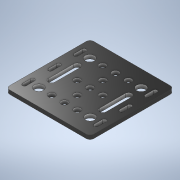
# Autodesk Inventor part: Plataforma
Saved by Autodesk Inventor 2021 (Build 250183000, 183)
## iProperties
Created: 2022-01-21
Part Number: Plataforma
Material: Generic
Document SubType Name: Modeling
Designer: deuts
Density: 1 g/cm^3
Appearance: Default
Author: deuts
Autodesk Inventor part; units mm, degrees
ref_plane "YZ Plane" through (0, 0, 0) normal (1, 0, 0) x (0, 1, 0)
ref_plane "XZ Plane" through (0, 0, 0) normal (0, 1, 0) x (-1, 0, 0)
ref_plane "XY Plane" through (0, 0, 0) normal (0, 0, 1) x (1, 0, 0)
sketch "Sketch1" plane through (0, 0, 0) normal (0, 1, 0) x (-1, 0, 0)
  line L0 (-29.75, 32.75) -> (29.75, 32.75)
  line L1 (32.75, 29.75) -> (32.75, -29.75)
  line L2 (29.75, -32.75) -> (-29.75, -32.75)
  line L3 (-32.75, -29.75) -> (-32.75, 29.75)
  arc A0 (-29.75, 32.75) -> (-32.75, 29.75) centre (-29.75, 29.75) ccw
  arc A1 (-32.75, -29.75) -> (-29.75, -32.75) centre (-29.75, -29.75) ccw
  arc A2 (29.75, -32.75) -> (32.75, -29.75) centre (29.75, -29.75) ccw
  arc A3 (32.75, 29.75) -> (29.75, 32.75) centre (29.75, 29.75) ccw
  arc A4 (29.2, 23.4) -> (26.2, 23.4) centre (27.7, 23.4) ccw
  arc A5 (26.2, 16.9) -> (29.2, 16.9) centre (27.7, 16.9) ccw
  line L4 (29.2, 23.4) -> (29.2, 16.9)
  line L5 (26.2, 23.4) -> (26.2, 16.9)
  arc A6 (29.2, 3.25) -> (26.2, 3.25) centre (27.7, 3.25) ccw
  arc A7 (26.2, -3.25) -> (29.2, -3.25) centre (27.7, -3.25) ccw
  line L6 (29.2, 3.25) -> (29.2, -3.25)
  line L7 (26.2, 3.25) -> (26.2, -3.25)
  circle A8 centre (20, 19.85) radius 3.6
  circle A9 centre (10, 19.85) radius 2.55
  circle A10 centre (0, 19.85) radius 2.55
  circle A11 centre (0, 10) radius 2.55
  circle A12 centre (0, 0) radius 2.55
  circle A13 centre (10, 0) radius 2.55
  arc A14 (22.5, 10) -> (17.5, 10) centre (20, 10) ccw
  arc A15 (17.5, -10) -> (22.5, -10) centre (20, -10) ccw
  line L8 (22.5, 10) -> (22.5, -10)
  line L9 (17.5, 10) -> (17.5, -10)
  circle A16 centre (-20, 19.85) radius 3.6
  circle A17 centre (20, -19.85) radius 3.6
  circle A18 centre (-20, -19.85) radius 3.6
  circle A19 centre (-10, 19.85) radius 2.55
  circle A20 centre (-10, -19.85) radius 2.55
  circle A21 centre (10, -19.85) radius 2.55
  circle A22 centre (0, -10) radius 2.55
  circle A23 centre (0, -19.85) radius 2.55
  circle A24 centre (-10, 0) radius 2.55
  arc A25 (-17.5, 10) -> (-22.5, 10) centre (-20, 10) ccw
  arc A26 (-22.5, -10) -> (-17.5, -10) centre (-20, -10) ccw
  line L10 (-17.5, 10) -> (-17.5, -10)
  line L11 (-22.5, 10) -> (-22.5, -10)
  arc A27 (29.2, -16.6) -> (26.2, -16.6) centre (27.7, -16.6) ccw
  arc A28 (26.2, -23.1) -> (29.2, -23.1) centre (27.7, -23.1) ccw
  line L12 (29.2, -16.6) -> (29.2, -23.1)
  line L13 (26.2, -16.6) -> (26.2, -23.1)
  line L14 (-32.75, 32.75) -> (-27.7, 32.75)
  arc A29 (-26.2, 23.1) -> (-29.2, 23.1) centre (-27.7, 23.1) ccw
  arc A30 (-29.2, 16.6) -> (-26.2, 16.6) centre (-27.7, 16.6) ccw
  line L15 (-26.2, 23.1) -> (-26.2, 16.6)
  line L16 (-29.2, 23.1) -> (-29.2, 16.6)
  arc A31 (-26.2, 3.25) -> (-29.2, 3.25) centre (-27.7, 3.25) ccw
  arc A32 (-29.2, -3.25) -> (-26.2, -3.25) centre (-27.7, -3.25) ccw
  line L17 (-26.2, 3.25) -> (-26.2, -3.25)
  line L18 (-29.2, 3.25) -> (-29.2, -3.25)
  arc A33 (-26.2, -16.6) -> (-29.2, -16.6) centre (-27.7, -16.6) ccw
  arc A34 (-29.2, -23.1) -> (-26.2, -23.1) centre (-27.7, -23.1) ccw
  line L19 (-26.2, -16.6) -> (-26.2, -23.1)
  line L20 (-29.2, -16.6) -> (-29.2, -23.1)
  point P0 (0, 0)
  point P1 (27.7, 0)
  point P2 (-27.7, 19.85)
  point P3 (-27.7, 0)
  point P4 (-27.7, -19.85)
  dimension "d2" = 3
  dimension "d7" = 3
  dimension "d8" = 3
  dimension "d10" = 3
  dimension "d12" = 3
  dimension "d16" = 7.2
  dimension "d18" = 5.1
  dimension "d20" = 5.1
  dimension "d22" = 5.1
  dimension "d23" = 5.1
  dimension "d24" = 5.1
  dimension "d26" = 5
  dimension "d28" = 5
  dimension "d31" = 10
  dimension "d36" = 7.2
  dimension "d39" = 29.5
  dimension "d44" = 7.2
  dimension "d45" = 7.2
  dimension "d46" = 5.1
  dimension "d47" = 5.1
  dimension "d48" = 5.1
  dimension "d51" = 5.1
  dimension "d52" = 5.1
  dimension "d53" = 5.1
  dimension "d54" = 5
  dimension "d55" = 5
  dimension "d56" = 3
  dimension "d57" = 3
  dimension "d58" = 5.05
  dimension "d59" = 3
  dimension "d60" = 3
  dimension "d61" = 3
  dimension "d62" = 3
  dimension "d63" = 3
  dimension "d64" = 3
  constraints: 42 end point, 40 point on circle, 35 centre point, 24 tangent, 5 parallel, 3 equal radius, 2 point on line, 1 horizontal, 1 perpendicular
  measures "d2" radius of A0
  measures "d7" diameter of A4
  measures "d8" diameter of A5
  measures "d10" diameter of A6
  measures "d12" diameter of A7
  measures "d16" diameter of A8
  measures "d18" diameter of A9
  measures "d20" diameter of A10
  measures "d22" diameter of A11
  measures "d23" diameter of A12
  measures "d24" diameter of A13
  measures "d26" diameter of A14
  measures "d28" diameter of A15
  measures "d31" distance of A9.centre A10.centre
  measures "d36" diameter of A16
  measures "d39" distance from line of L0 A6.centre
  measures "d44" diameter of A17
  measures "d45" diameter of A18
  measures "d46" diameter of A19
  measures "d47" diameter of A20
  measures "d48" diameter of A21
  measures "d51" diameter of A22
  measures "d52" diameter of A23
  measures "d53" diameter of A24
  measures "d54" diameter of A25
  measures "d55" diameter of A26
  measures "d56" diameter of A27
  measures "d57" diameter of A28
  measures "d58" distance of L14.start L14.end
  measures "d59" diameter of A29
  measures "d60" diameter of A30
  measures "d61" diameter of A31
  measures "d62" diameter of A32
  measures "d63" diameter of A33
  measures "d64" diameter of A34
extrude "Extrusion1" add sketch "Sketch1" along normal blind 3
body "Solid1"
